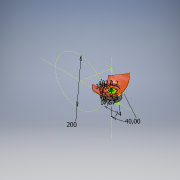
# Autodesk Inventor part: HarmonicDrive3
Saved by Autodesk Inventor 2018.3 (Build 223284000, 284)
## iProperties
Created: 2018-07-04
Part Number: HarmonicDrive3
Material: Generisch
Document SubType Name: Modeling
Designer: JochenAlt
Density: 1 g/cm^3
Appearance: Vorgabe
Author: JochenAlt
Autodesk Inventor part; units mm, degrees
ref_plane "YZ Plane" through (0, 0, 0) normal (1, 0, 0) x (0, 1, 0)
ref_plane "XZ Plane" through (0, 0, 0) normal (0, 1, 0) x (-1, 0, 0)
ref_plane "XY Plane" through (0, 0, 0) normal (0, 0, 1) x (1, 0, 0)
sketch "Skizze4" plane through (0, 0, 0) normal (0, 0, 1) x (1, 0, 0)
  circle A0 centre (0, 0) radius 3
  circle A1 centre (0, 0) radius 5.15
  circle A2 centre (0, 0) radius 6.65
  circle A3 centre (0, 0) radius 4.15
  line L0 (-295.2103, 0) -> (112.2621, 0) construction
  line L1 (0, -9.31) -> (0, 9.31) construction
  dimension "d25" = 6
  dimension "d26" = 10.3
  dimension "d27" = 1.5
  dimension "d28" = 1
  constraints: 4 centre point, 4 coincident
  measures "d25" diameter of A0
  measures "d26" diameter of A1
  measures "d27" radial gap between concentric circles of A2 A1
  measures "d28" radial gap between concentric circles of A1 A3
extrude "Extrusion4" add sketch "Skizze4" along normal blind 2 contours A1 | A2 | A3
extrude "Extrusion5" add sketch "Skizze4" along normal blind 3 from surface at 2 contours A2
extrude "Extrusion6" add sketch "Skizze4" along normal blind 0.5 from surface at 2 contours A1
sketch "Skizze5" plane through (0, 0, 0) normal (0, 1, 0) x (-1, 0, 0)
  line L0 (37, -5) -> (-37, -5) construction
  line L1 (0, -22.142) -> (0, 36.357) construction
  circle A0 centre (28.215, -5) radius 8.785 construction
  circle A1 centre (-28.215, -5) radius 8.785 construction
  line L2 (-6.65, 0) -> (6.65, 0) construction
  line L3 (6.65, 0) -> (6.65, 5) construction
  arc A2 (32.1364, 5.0468) -> (18.9324, 0.4909) centre (28.215, -5) ccw
  line L4 (18.0717, 0) -> (6.65, 0)
  line L5 (33.5, 5.9784) -> (33.5, 30)
  line L6 (31.5, 8.5943) -> (31.5, 28)
  line L7 (6.65, 2) -> (16.9889, 2)
  line L8 (6.65, 2) -> (6.65, 0)
  arc A3 (30.3342, 7.6081) -> (17.8032, 2.4197) centre (28.215, -5) ccw
  line L9 (33.5, 30) -> (29.5, 30)
  line L10 (29.5, 30) -> (29.5, 28)
  line L11 (29.5, 28) -> (31.5, 28)
  arc A4 (18.0717, 0) -> (18.9324, 0.4909) centre (18.0717, 1) ccw
  arc A5 (16.9889, 2) -> (17.8032, 2.4197) centre (16.9889, 3) ccw
  arc A6 (30.3342, 7.6081) -> (31.5, 8.5943) centre (30.5, 8.5943) ccw
  arc A7 (32.1364, 5.0468) -> (33.5, 5.9784) centre (32.5, 5.9784) ccw
  circle A8 centre (137, -5) radius 100 construction
  line L12 (137, -5) -> (0, 109.9566) construction
  line L13 (0, 109.9566) -> (-54.0517, 45.5403) construction
  line L14 (33.5, 30) -> (33.5, 40) construction
  line L15 (33.5, 40) -> (-33.5, 40) construction
  line L16 (33.5, 30) -> (-33.5, 30) construction
  line L17 (-33.5, 30) -> (-33.5, 40) construction
  line L18 (-33.5, 30) -> (-33.5, 32.173)
  line L19 (33.5, 30) -> (33.5, 32.173)
  arc A9 (-33.5, 32.173) -> (33.5, 32.173) centre (0, 109.9566) ccw
  arc A10 (-33.5, 30) -> (33.5, 30) centre (0, 109.9566) ccw
  line L20 (0, -147.9913) -> (0, 152.948) construction
  line L21 (295.2103, 0) -> (-112.2621, 0) construction
  point P0 (0, 0)
  point P1 (0, 0)
  point P2 (33.5, 4.4013)
  point P3 (18.659, 0)
  point P4 (31.5, 7.3558)
  point P5 (17.5166, 2)
  dimension "d32" = 17.57
  dimension "d31" = 74
  dimension "d33" = 5
  dimension "d34" = 2
  dimension "d35" = 2
  dimension "d36" = 2
  dimension "d37" = 2
  dimension "d38" = 33.5
  dimension "d39" = 30
  dimension "d40" = 1
  dimension "d41" = 4
  dimension "d42" = 200
  dimension "d43" = 40
  dimension "d44" = 10
  dimension "d45" = 2
  constraints: 40 end point, 20 point on circle, 10 point on line, 9 centre point, 8 tangent, 5 horizontal, 4 coincident, 4 perpendicular, 4 vertical, 3 equal radius, 2 collinear, 2 horizontal alignment, 1 parallel, 1 symmetric about line, 7 other
  measures "d31" distance of L0.end L0.start
  measures "d33" distance between parallel lines of L0 L2
  measures "d35" distance between parallel lines of L4 L7
  measures "d36" radial gap between concentric circles of A3 A2
  measures "d37" distance between parallel lines of L6 L5
  measures "d38" distance between parallel lines of L5 L1
  measures "d39" distance between parallel lines of L9 L4
  measures "d40" radius of A4
  measures "d41" distance of L5.end L9.end
  measures "d42" diameter of A8
  measures "d43" angle of L13 L1
  measures "d44" distance of L5.end L14.end
  measures "d45" radial gap between concentric circles of A9 A10
revolve "Umdrehung1" add sketch "Skizze5" angle 360 about axis through (0, 0, -22.142) along (0, 0, 1) contours A2 A4 L4 L8 L7 A5 A3 A6 L6 L11 L10 A10 L5 A7 | A10 L10 L9
ref_plane "Arbeitsebene1" through (0, 0, 8) normal (0, 0, 1) x (1, 0, 0)
sketch "Skizze6" plane through (0, 0, 8) normal (0, 0, 1) x (1, 0, 0)
  line L0 (0, 0) -> (-30.3613, 14.1577)
  line L1 (0, 0) -> (-14.1577, 30.3613)
  line L2 (0, 0) -> (14.1577, 30.3613)
  line L3 (0, 0) -> (14.1577, -30.3613)
  line L4 (0, 0) -> (-14.1577, -30.3613)
  line L5 (0, 0) -> (-30.3613, -14.1577)
  arc A0 (14.1577, 30.3613) -> (-14.1577, 30.3613) centre (0, 0) ccw
  arc A1 (-30.3613, 14.1577) -> (-30.3613, -14.1577) centre (0, 0) ccw
  arc A2 (-14.1577, -30.3613) -> (14.1577, -30.3613) centre (0, 0) ccw
  line L6 (-9.4506, 0) -> (22.5494, 0)
  circle A3 centre (0, 0) radius 33.5 construction
  line L7 (-46.9, 0) -> (46.9, 0) construction
  line L8 (0, -50.1278) -> (0, 50.1278) construction
  line L9 (0, 16) -> (29.4321, 16)
  line L10 (29.4321, -16) -> (0, -16)
  line L11 (0, 16) -> (0, -16)
  arc A4 (29.4321, -16) -> (29.4321, 16) centre (0, 0) ccw
  dimension "d52" = 50
  dimension "d71" = 50
  dimension "d73" = 32
  constraints: 20 end point, 8 point on circle, 4 centre point, 3 point on line, 2 coincident, 2 concentric, 2 perpendicular, 1 collinear, 1 horizontal, 9 other
  measures "d52" angle of L2 L1
  measures "d71" angle of L5 L0
  measures "d73" distance between parallel lines of L10 L9
extrude "Extrusion7" cut sketch "Skizze6" along normal blind 19
fillet "Rundung1" radius 9.5 12 edges at (13.6937, 29.3663, 8) (-13.6937, 29.3663, 8) (-13.7351, 29.455, 27) (13.7351, 29.455, 27) (-29.455, 13.7351, 27) (-29.455, -13.7351, 27) (-29.3663, 13.6937, 8) (-29.3663, -13.6937, 8) (-13.6937, -29.3663, 8) (13.6937, -29.3663, 8) (13.7351, -29.455, 27) (-13.7351, -29.455, 27)
sketch "Skizze7" plane through (0, 0, 30) normal (0, 0, 1) x (1, 0, 0)
  circle A0 centre (0, 0) radius 29.3
  circle A1 centre (0, 0) radius 6.65
  circle A2 centre (0, 0) radius 5.15
  circle A3 centre (0, 0) radius 4.15
  circle A4 centre (0, 0) radius 3
  circle A5 centre (0, 0) radius 9.75
  circle A6 centre (0, 0) radius 11.75
  circle A7 centre (0, 0) radius 33.5 projected
  circle A8 centre (0, 0) radius 29.5 construction
  line L0 (0, -46.9) -> (0, 46.9) construction
  line L1 (-46.9, 0) -> (46.9, 0) construction
  circle A9 centre (0, 0) radius 31.5
  circle A10 centre (0, 0) radius 27.3
  dimension "d60" = 2
  dimension "d64" = 2
  dimension "d65" = 2
  dimension "d68" = 0.2
  constraints: 9 centre point, 5 coincident
  measures "d60" radial gap between concentric circles of A6 A5
  measures "d64" radial gap between concentric circles of A9 A7
  measures "d65" radial gap between concentric circles of A0 A10
  measures "d68" radial gap between concentric circles of A0 A8
extrude "Extrusion8" add sketch "Skizze7" against normal blind 2 separate body contours A0 | A6 | A10
extrude "Extrusion9" add sketch "Skizze7" along normal blind 2 contours A0 | A7 | A9 bodies 2
revolve "Umdrehung2" add sketch "Skizze5" angle 120 mid plane about axis through (-137, 0, -5) along (0.7660444, 0, 0.6427876) separate body contours A10 L10 L9 | L9 L10 A10 L18 A9 L19
extrude "Extrusion10" cut sketch "Skizze7" along normal through all both and the other way through all contours A0 | A1 | A2 | A3 | A4 | A5 | A6 | A7 | A9 | A10 bodies 3
combine bodies "Kombinieren1" operation type add bodies to combine 2 3
equation "\"d36\" = d35"
equation "\"d37\" = d35"
equation "\"d71\" = d52"
